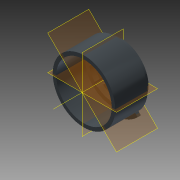
# Autodesk Inventor part: motor_GM1806-80T_SkyproRO_stator
Saved by Autodesk Inventor 2015 SP1 (Build 190203100, 203)
## iProperties
Created: 2015-08-06
Part Number: motor_GM1806-80T_SkyproRO_stator
Material: Iron, Cast
Document SubType Name: Modeling
Designer: Alexandre Cherpillod
Density: 7.15 g/cm^3
Appearance: Iron Gray
Mass: 10.9032 g
Surface Area: 25.758 cm^2
Volume: 1.52492 cm^3
Author: Alexandre Cherpillod
Autodesk Inventor part; units mm, degrees
ref_plane "XZ Plane" through (0, 0, 0) normal (0, 1, 0) x (-1, 0, 0)
sketch "Sketch1" plane through (0, 0, 0) normal (0, 1, 0) x (-1, 0, 0)
  circle A0 centre (0, 0) radius 11.5
  dimension "d0" = 23
  constraints: 1 centre point, 1 coincident
  measures "d0" diameter of A0
extrude "Extrusion1" add sketch "Sketch1" along normal blind 11.9
sketch "Sketch2" plane through (0, 11.9, 0) normal (0, 1, 0) x (1, 0, 0)
  circle A0 centre (0, 0) radius 10
  dimension "d3" = 20
  constraints: 1 centre point, 1 coincident
  measures "d3" diameter of A0
extrude "Extrusion2" add sketch "Sketch2" along normal blind 1.85
sketch "Sketch3" plane through (0, 13.75, 0) normal (0, 1, 0) x (1, 0, 0)
  circle A0 centre (0, 0) radius 10 projected
  circle A1 centre (0, 6.5) radius 2.5
  dimension "d6" = 5
  dimension "d23" = 6.5
  constraints: 1 centre point
  measures "d6" diameter of A1
  measures "d23" distance of point (0, 0) A1.centre
extrude "Extrusion3" cut sketch "Sketch3" against normal blind 5 contours A1
ref_plane "Work Plane1" through (0, 0, 0) normal (0.7071068, 0, 0.7071068) x (0, 1, 0)
sketch "Sketch4" plane through (0, 13.75, 0) normal (0, 1, 0) x (1, 0, 0)
  line L0 (16.1, 16.1) -> (-16.1, -16.1) projected
  point P0 (0, 0)
  point P1 (5.6569, 5.6569)
  dimension "d10" = 8
  constraints: 1 point on line
  measures "d10" distance of point (0, 0) point (5.657, 5.657)
hole "Hole1" at (5.6569, 13.75, -5.6569) direction (0, -1, 0) diameter 2 depth 4.5 tip angle 118
pattern_circular "Circular Pattern1" count 4 over 360 about axis through (0, -10, 0) along (0, 1, 0) of "Extrusion3", "Hole1"
shell "Shell1" thickness 1.3 removed faces 17 at (-0.1507, 0, 2.542) at (-0.852, 8.75, -7.0526) at (6.099, 10.4167, 2.4676) at (7.0526, 8.75, -0.852) at (2.4676, 10.4167, -6.099) at (5.7373, 12.25, -4.6601) at (5.843, 9.1165, -4.9017) at (6.3455, 9.1165, 6.0183) at (4.6601, 12.25, 5.7373) at (0.852, 8.75, 7.0526) at (-2.4676, 10.4167, 6.099) at (-7.0526, 8.75, 0.852) at (-6.099, 10.4167, -2.4676) at (-5.843, 9.1165, 4.9017) at (-5.7373, 12.25, 4.6601) at (-4.9017, 9.1165, -5.843) at (-4.6601, 12.25, -5.7373)
sketch "Sketch5" plane through (0, 11.9, 0) normal (0, 1, 0) x (1, 0, 0)
  arc A0 (9.0498, 9.0605) -> (-8.5529, 9.531) centre (0, 0) ccw
  arc A1 (8.1423, 8.1211) -> (-7.76, 8.4872) centre (0, 0) ccw
  line L0 (-8.5529, 9.531) -> (-7.76, 8.4872)
  line L1 (8.1423, 8.1211) -> (9.0498, 9.0605)
  constraints: 4 end point, 4 point on circle, 2 centre point, 2 coincident
extrude "Extrusion4" add sketch "Sketch5" against normal blind 1.2
body "Solid1"
